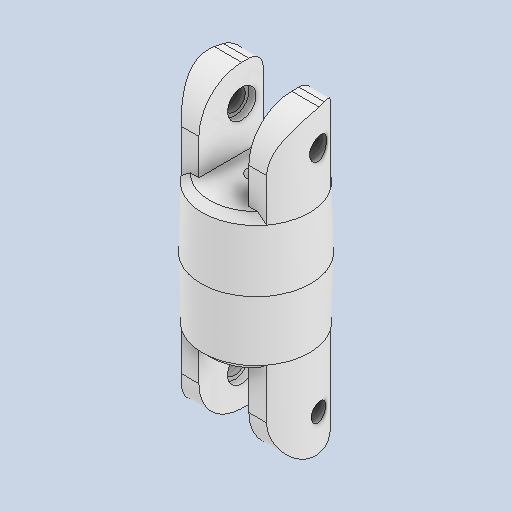
# Autodesk Inventor part: Lil_1
Saved by Autodesk Inventor 2022 (Build 260153000, 153)
## iProperties
Created: 2023-01-15
Part Number: Lil_1
Material: ABS Plastic
Document SubType Name: Modeling
Designer: 48735
Density: 1.06 g/cm^3
Appearance: Smooth - White
Author: 48735
Autodesk Inventor part; units mm, degrees
ref_plane "YZ Plane" through (0, 0, 0) normal (1, 0, 0) x (0, 1, 0)
ref_plane "XZ Plane" through (0, 0, 0) normal (0, 1, 0) x (-1, 0, 0)
ref_plane "XY Plane" through (0, 0, 0) normal (0, 0, 1) x (1, 0, 0)
sketch "Sketch1" plane through (0, 0, 0) normal (0, 1, 0) x (-1, 0, 0)
  circle A0 centre (0, 0) radius 7.5
  line L0 (0, 0) -> (3.5, 0)
  line L1 (3.5, 0) -> (-3.5, 0)
  line L2 (-3.5, 0) -> (-3.5, -3.5)
  line L3 (-3.5, 0) -> (-3.5, 3.5)
  line L4 (3.5, 0) -> (3.5, -3.5)
  line L5 (3.5, 0) -> (3.5, 3.5)
  line L6 (3.5, -3.5) -> (3.5, -4.5)
  line L7 (3.5, -4.5) -> (6, -4.5)
  line L8 (3.5, 3.5) -> (3.5, 4.5)
  line L9 (3.5, 4.5) -> (6, 4.5)
  line L10 (-3.5, 3.5) -> (-3.5, 4.5)
  line L11 (-3.5, 4.5) -> (-6, 4.5)
  line L12 (-3.5, -3.5) -> (-3.5, -4.5)
  line L13 (-3.5, -4.5) -> (-6, -4.5)
  point P0 (-6.6332, -3.5)
  point P1 (-6.6332, 3.5)
  point P2 (6.6332, -3.5)
  point P3 (6.6332, 3.5)
  constraints: 28 end point, 8 point on line, 3 perpendicular, 1 coincident, 1 horizontal, 1 vertical, 10 other
extrude "Extrusion1" add sketch "Sketch1" along normal blind 12 contours A0 L7 L6 L4 L5 L8 L9 | L11 L10 L3 L2 L12 L13 A0
sketch "Sketch2" plane through (0, 12, 0) normal (0, 1, 0) x (1, 0, 0)
  circle A0 centre (0, 0) radius 7.5
  circle A1 centre (0, 0) radius 1.25
  dimension "d7" = 2.5
  constraints: 2 centre point, 2 coincident
  measures "d7" diameter of A1
extrude "Extrusion2" add sketch "Sketch2" along normal blind 1
fillet "Fillet1" radius 6 2 edges at (-4.75, 0, 4.5) (4.75, 0, 4.5)
fillet "Fillet2" radius 2 2 edges at (-4.75, 0, -4.5) (4.75, 0, -4.5)
sketch "Sketch3" plane through (3.5, 12, -4.5) normal (-1, 0, 0) x (0, 0, 1)
  arc A0 (3, -12) -> (9, -6) centre (3, -6) ccw projected
  line L0 (3, -12) -> (3, -7)
  point P0 (4.5, -12)
  dimension "d16" = 5
  constraints: 2 end point, 1 vertical
  measures "d16" distance of L0.start L0.end
hole "Hole1" at (3.5, 5, -1.5) direction (1, 0, 0) diameter 2.5 depth 5 counterbore diameter 4 counterbore depth 1
sketch "Sketch4" plane through (-3.5, 12, 4.5) normal (1, 0, 0) x (0, 0, -1)
  line L0 (6, -12) -> (7, -12) projected
  line L1 (6, -12) -> (6, -7)
  point P0 (4.5, -12)
  dimension "d24" = 5
  constraints: 2 end point, 1 vertical
  measures "d24" distance of L0.start L1.end
hole "Hole2" at (-3.5, 5, -1.5) direction (-1, 0, 0) diameter 3 depth 5 counterbore diameter 4 counterbore depth 1
sketch "Sketch5" plane through (0, 13, 0) normal (0, 1, 0) x (1, 0, 0)
  circle A0 centre (0, 0) radius 1.25
  circle A1 centre (0, 0) radius 1.25 projected
  circle A2 centre (0, 0) radius 7.7
  dimension "d32" = 15.4
  constraints: 2 centre point, 2 coincident
  measures "d32" diameter of A2
extrude "Extrusion3" add sketch "Sketch5" along normal blind 8.5
chamfer "Chamfer1" distance 8.5 distance2 0.2 1 edges at (-7.7, 13, 0) measured on face at (7.6003, 18.6667, 1.2352)
sketch "Sketch6" plane through (0, 21.5, 0) normal (0, 1, 0) x (1, 0, 0)
  circle A0 centre (0, 0) radius 1.25
  circle A1 centre (0, 0) radius 7.7
  constraints: 2 centre point, 2 coincident
extrude "Extrusion4" add sketch "Sketch6" along normal blind 8.5
chamfer "Chamfer2" distance 0.2 distance2 8.5 1 edges at (-7.7, 30, 0) measured on face at (5.4633, 30, 0.714)
sketch "Sketch7" plane through (0, 30, 0) normal (0, 1, 0) x (1, 0, 0)
  circle A0 centre (0, 0) radius 1.25
  circle A1 centre (0, 0) radius 1.25 projected
  circle A2 centre (0, 0) radius 7.5
  constraints: 2 centre point, 2 coincident
extrude "Extrusion5" add sketch "Sketch7" along normal blind 1
chamfer "Chamfer3" distance 1 angle 45 2 edges at (0, 12, 7.5) (0, 12, -7.5)
fillet "Fillet3" radius 1 1 edges at (-1.25, 12, 0)
sketch "Sketch8" plane through (0, 31, 0) normal (0, 1, 0) x (1, 0, 0)
  circle A0 centre (0, 0) radius 7.5
  line L0 (0, 0) -> (3.5, 0)
  line L1 (3.5, 0) -> (-3.5, 0)
  line L2 (-3.5, 0) -> (-3.5, -3.5)
  line L3 (-3.5, 0) -> (-3.5, 3.5)
  line L4 (3.5, 0) -> (3.5, -3.5)
  line L5 (3.5, 0) -> (3.5, 3.5)
  line L6 (3.5, -3.5) -> (3.5, -4.5)
  line L7 (3.5, -4.5) -> (6, -4.5)
  line L8 (3.5, 3.5) -> (3.5, 4.5)
  line L9 (3.5, 4.5) -> (6, 4.5)
  line L10 (-3.5, 3.5) -> (-3.5, 4.5)
  line L11 (-3.5, 4.5) -> (-6, 4.5)
  line L12 (-3.5, -3.5) -> (-3.5, -4.5)
  line L13 (-3.5, -4.5) -> (-6, -4.5)
  point P0 (-6.6332, -3.5)
  point P1 (-6.6332, 3.5)
  point P2 (6.6332, -3.5)
  point P3 (6.6332, 3.5)
  constraints: 28 end point, 8 point on line, 3 perpendicular, 1 coincident, 1 horizontal, 1 vertical, 10 other
extrude "Extrusion6" add sketch "Sketch8" along normal blind 11 contours A0 L7 L6 L4 L5 L8 L9 | L11 L10 L3 L2 L12 L13 A0
fillet "Fillet4" radius 6 2 edges at (4.75, 42, 4.5) (-4.75, 42, 4.5)
fillet "Fillet5" radius 2 2 edges at (4.75, 42, -4.5) (-4.75, 42, -4.5)
sketch "Sketch9" plane through (3.5, 31, -4.5) normal (-1, 0, 0) x (0, 0, 1)
  line L0 (2, 11) -> (3, 11) projected
  line L1 (3, 11) -> (3, 6)
  point P0 (4.5, -31)
  dimension "d54" = 5
  constraints: 2 end point, 1 vertical
  measures "d54" distance of L0.end L1.end
hole "Hole3" at (3.5, 37, -1.5) direction (1, 0, 0) diameter 3 depth 5 counterbore diameter 4 counterbore depth 1
sketch "Sketch10" plane through (-3.5, 31, 4.5) normal (1, 0, 0) x (0, 0, -1)
  arc A0 (6, 11) -> (0, 5) centre (6, 5) ccw projected
  line L0 (6, 11) -> (6, 6)
  point P0 (4.5, -31)
  dimension "d62" = 5
  constraints: 2 end point, 1 vertical
  measures "d62" distance of L0.start L0.end
hole "Hole4" at (-3.5, 37, -1.5) direction (-1, 0, 0) diameter 3 depth 5 counterbore diameter 4 counterbore depth 1
chamfer "Chamfer4" distance 1 angle 45 2 edges at (0, 31, 7.5) (0, 31, -7.5)
thread "Thread1" size "M2.5x0.45" class "6H" standard "ANSI Metric M Profile" length 6
thread "Thread2" size "M3x0.5" class "6H" standard "ANSI Metric M Profile" length 6
thread "Thread3" size "M3x0.5" class "6H" standard "ANSI Metric M Profile" length 6
thread "Thread4" size "M3x0.5" class "6H" standard "ANSI Metric M Profile" length 6
body "Solid1"
